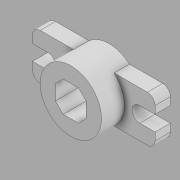
# Autodesk Inventor part: Lab2A01209499P10
Saved by Autodesk Inventor 2020 (Build 240168000, 168)
## iProperties
Created: 2019-08-22
Part Number: Lab2A01209499P10
Material: Genérico
Document SubType Name: Modeling
Designer: gerar
Density: 1 g/cm^3
Appearance: Valor por defecto
Author: gerar
Autodesk Inventor part; units mm, degrees
ref_plane "YZ Plane" through (0, 0, 0) normal (1, 0, 0) x (0, 1, 0)
ref_plane "XZ Plane" through (0, 0, 0) normal (0, 1, 0) x (-1, 0, 0)
ref_plane "XY Plane" through (0, 0, 0) normal (0, 0, 1) x (1, 0, 0)
sketch "Boceto1" plane through (0, 0, 0) normal (0, 0, 1) x (1, 0, 0)
  line L0 (-80, -30) -> (80, -30)
  line L1 (80, 30) -> (-80, 30)
  line L2 (-80, -30) -> (80, 30) construction
  line L3 (80, -30) -> (-80, 30) construction
  line L4 (0, -42) -> (0, 42) construction
  line L5 (-112, 0) -> (112, 0) construction
  arc A0 (-60, -10) -> (-60, 10) centre (-60, 0) ccw
  line L6 (-80, 10) -> (-60, 10)
  line L7 (-80, -10) -> (-60, -10)
  arc A1 (60, 10) -> (60, -10) centre (60, 0) ccw
  line L8 (80, 10) -> (60, 10)
  line L9 (80, -10) -> (60, -10)
  line L10 (-80, 30) -> (-80, 10)
  line L11 (-80, -10) -> (-80, -30)
  line L12 (80, -30) -> (80, -10)
  line L13 (80, 10) -> (80, 30)
  point P0 (0, 0)
  dimension "d2" = 160
  dimension "d3" = 60
  dimension "d4" = 20
  dimension "d6" = 20
  dimension "d7" = 20
  constraints: 24 end point, 6 parallel, 5 symmetric about line, 4 point on circle, 3 horizontal, 2 centre point, 2 midpoint, 2 perpendicular, 2 tangent, 1 point on line, 1 other
  measures "d2" distance of L1.end L1.start
  measures "d3" distance of L1.start L0.end
  measures "d4" diameter of A0
  measures "d6" distance from line of L11 A0.centre
  measures "d7" distance from line of L12 A1.centre
extrude "Extrusión1" add sketch "Boceto1" along normal blind 20
sketch "Boceto2" plane through (0, 0, 20) normal (0, 0, 1) x (1, 0, 0)
  circle A0 centre (0, 0) radius 40
  dimension "d10" = 80
  constraints: 1 centre point, 1 coincident
  measures "d10" diameter of A0
extrude "Extrusión2" add sketch "Boceto2" along normal blind 30 and the other way blind 20
sketch "Boceto3" plane through (0, 0, 50) normal (0, 0, 1) x (1, 0, 0)
  line L0 (-10, -20) -> (10, -20)
  line L1 (20, -10) -> (20, 10)
  line L2 (10, 20) -> (-10, 20)
  line L3 (-20, 10) -> (-20, -10)
  line L4 (-20, -20) -> (20, 20) construction
  line L5 (20, -20) -> (-20, 20) construction
  line L6 (-10, 20) -> (-20, 10)
  line L7 (10, 20) -> (20, 10)
  line L8 (20, -10) -> (10, -20)
  line L9 (-10, -20) -> (-20, -10)
  point P0 (0, 0)
  dimension "d15" = 40
  dimension "d16" = 40
  dimension "d17" = 10
  dimension "d18" = 10
  dimension "d19" = 10
  dimension "d20" = 10
  dimension "d21" = 10
  dimension "d22" = 10
  dimension "d23" = 10
  dimension "d24" = 10
  constraints: 20 end point, 8 point on line, 2 midpoint, 2 parallel, 1 horizontal, 1 perpendicular
  measures "d15" distance of L5.end L4.end
  measures "d16" distance of L4.end L5.start
  measures "d17" distance of L2.end L5.end
  measures "d18" distance of L3.start L5.end
  measures "d19" distance of L2.start L4.end
  measures "d20" distance of L1.end L4.end
  measures "d21" distance of L1.start L5.start
  measures "d22" distance of L0.end L5.start
  measures "d23" distance of L0.start L4.start
  measures "d24" distance of L3.end L4.start
extrude "Extrusión3" cut sketch "Boceto3" against normal through all
fillet "Empalme1" radius 10 4 edges at (80, 30, 10) (-80, 30, 10) (80, -30, 10) (-80, -30, 10)
equation "\"d18\" = d17"
equation "\"d19\" = d17"
equation "\"d20\" = d19"
equation "\"d21\" = d17"
equation "\"d22\" = d21"
equation "\"d23\" = d17"
equation "\"d24\" = d23"
